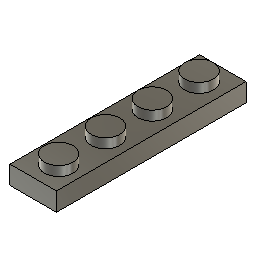
R4xC1xT3_1 (Autodesk Fusion 360 design; units mm, degrees)
Autodesk Fusion 360 part; units mm, degrees
sketch "Sketch1" plane through (0, 0, 0) normal (0, 0, 1) x (1, 0, 0)
  line L0 (0, 0) -> (7.8, 0)
  line L1 (7.8, 0) -> (7.8, 31.8)
  line L2 (7.8, 31.8) -> (0, 31.8)
  line L3 (0, 31.8) -> (0, 0)
  dimension "d1" = 7.8
  dimension "d2" = 31.8
  constraint horizontal L0
  constraint vertical L1
  constraint horizontal L2
  constraint vertical L3
  constraint coincident L0.start L3.end
  measures "d1" distance of L1.end L2.end
  measures "d2" distance of L0.end L1.end
extrude "Extrude1" add sketch "Sketch1" along normal blind 3.1
sketch "Sketch2" plane through (0, 0, 0) normal (0, 0, -1) x (1, 0, 0)
  line L0 (0, 0) -> (0, -31.8)
  line L1 (0, -31.8) -> (7.8, -31.8)
  line L2 (7.8, -31.8) -> (7.8, 0)
  line L3 (7.8, 0) -> (0, 0)
  line L4 (1.4, -1.4) -> (6.4, -1.4)
  line L5 (6.4, -1.4) -> (6.4, -30.4)
  line L6 (6.4, -30.4) -> (1.4, -30.4)
  line L7 (1.4, -30.4) -> (1.4, -1.4)
  dimension "d5" = 1.4
  dimension "d6" = 1.4
  dimension "d7" = 1.4
  dimension "d8" = 1.4
  constraint horizontal L4
  constraint vertical L5
  constraint horizontal L6
  constraint vertical L7
  measures "d5" distance of L0 L7
  measures "d6" distance of L3 L4
  measures "d7" distance of L1 L6
  measures "d8" distance of L2 L5
extrude "Extrude2" cut sketch "Sketch2" against normal blind 2 contours L4 L5 L6 L7
sketch "Sketch3" plane through (0, 0, 3.1) normal (0, 0, 1) x (-1, 0, 0)
  line L0 (0, -31.8) -> (0, 0)
  line L1 (0, 0) -> (-7.8, 0)
  line L2 (-7.8, 0) -> (-7.8, -31.8)
  line L3 (-7.8, -31.8) -> (0, -31.8)
  circle A0 centre (-3.9, -27.825) radius 2.4
  circle A1 centre (-3.997, -19.875) radius 2.4
  circle A2 centre (-4.0941, -11.925) radius 2.4
  circle A3 centre (-4.1911, -3.975) radius 2.4
  dimension "d11" = 4.8
  dimension "d12" = 4.8
  dimension "d13" = 4.8
  dimension "d14" = 4.8
  dimension "d15" = 3.9
  dimension "d16" = 7.95
  dimension "d17" = 7.95
  dimension "d18" = 7.95
  dimension "d19" = 3.975
  constraint collinear A0.centre A1.centre A2.centre
  constraint collinear A0.centre A1.centre A3.centre
  measures "d11" diameter of A0
  measures "d12" diameter of A1
  measures "d13" diameter of A2
  measures "d14" diameter of A3
  measures "d15" distance of L0 A0.centre
  measures "d16" vertical distance of A2.centre A3.centre
  measures "d17" vertical distance of A1.centre A2.centre
  measures "d18" vertical distance of A0.centre A1.centre
  measures "d19" distance of L1 A3.centre
extrude "Extrude3" add sketch "Sketch3" along normal blind 1.6 contours A0 | A1 | A2 | A3
sketch "Sketch4" plane through (0, 0, 2) normal (0, 0, -1) x (1, 0, 0)
  line L0 (1.4, -30.4) -> (6.4, -30.4)
  line L1 (6.4, -30.4) -> (6.4, -1.4)
  line L2 (6.4, -1.4) -> (1.4, -1.4)
  line L3 (1.4, -1.4) -> (1.4, -30.4)
  circle A0 centre (3.9, -7.95) radius 1.45
  circle A1 centre (3.9, -15.9) radius 1.45
  circle A2 centre (3.9, -23.85) radius 1.45
  circle A3 centre (3.9, -7.95) radius 0.75
  circle A4 centre (3.9, -15.9) radius 0.75
  circle A5 centre (3.9, -23.85) radius 0.75
  dimension "d22" = 2.9
  dimension "d23" = 2.9
  dimension "d24" = 2.9
  dimension "d28" = 7.95
  dimension "d29" = 7.95
  dimension "d30" = 7.95
  dimension "d31" = 3.9
  dimension "d32" = 1.5
  dimension "d33" = 1.5
  dimension "d34" = 1.5
  constraint collinear A0.centre A1.centre A2.centre
  constraint concentric A0 A3
  constraint concentric A1 A4
  constraint concentric A2 A5
  measures "d22" diameter of A0
  measures "d23" diameter of A1
  measures "d24" diameter of A2
  measures "d28" vertical distance of A0.centre origin
  measures "d29" distance of A0.centre A1.centre
  measures "d30" distance of A1.centre A2.centre
  measures "d31" horizontal distance of A0.centre origin
  measures "d32" diameter of A3
  measures "d33" diameter of A4
  measures "d34" diameter of A5
extrude "Extrude4" add sketch "Sketch4" along normal blind 2 contours A0 | A1 | A2
